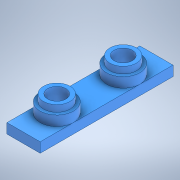
# Autodesk Inventor part: 4mm_Roller_Spacer
Saved by Autodesk Inventor 2021 (Build 250183000, 183)
## iProperties
Created: 2021-03-29
Part Number: 4mm_Roller_Spacer
Material: PET Plastic
Document SubType Name: Modeling
Designer: Jorian Brusind
Density: 1.541 g/cm^3
Appearance: Cyan
Author: Jorian Brusind
Autodesk Inventor part; units mm, degrees
ref_plane "YZ Plane" through (0, 0, 0) normal (1, 0, 0) x (0, 1, 0)
ref_plane "XZ Plane" through (0, 0, 0) normal (0, 1, 0) x (-1, 0, 0)
ref_plane "XY Plane" through (0, 0, 0) normal (0, 0, 1) x (1, 0, 0)
sketch "Sketch1" plane through (0, 0, 0) normal (0, 1, 0) x (-1, 0, 0)
  line L0 (0, 0) -> (10, 0)
  line L1 (10, 0) -> (10, -40)
  line L2 (10, -40) -> (0, -40)
  line L3 (0, -40) -> (0, 0)
  circle A0 centre (5, -10) radius 2.75
  circle A1 centre (5, -30) radius 2.75
  dimension "d0" = 10
  dimension "d1" = 40
  dimension "d2" = 5.5
  dimension "d3" = 5.5
  dimension "d4" = 10
  dimension "d5" = 10
  dimension "d6" = 5
  constraints: 8 end point, 2 centre point, 2 parallel, 1 horizontal, 1 perpendicular, 1 vertical alignment
  measures "d0" distance of L1.end L2.end
  measures "d1" distance of L0.end L1.end
  measures "d2" diameter of A0
  measures "d3" diameter of A1
  measures "d4" distance from line of L2 A1.centre
  measures "d5" distance from line of L0 A0.centre
  measures "d6" distance from line of L1 A0.centre
extrude "Extrusion1" add sketch "Sketch1" along normal blind 3
sketch "Sketch2" plane through (0, 3, 0) normal (0, 1, 0) x (1, 0, 0)
  circle A0 centre (-5, 10) radius 2.75 projected
  circle A1 centre (-5, 10) radius 2.75
  circle A2 centre (-5, 10) radius 4
  circle A3 centre (-5, 30) radius 2.75 projected
  circle A4 centre (-5, 30) radius 2.75
  circle A5 centre (-5, 30) radius 4
  point P0 (0, 0)
  dimension "d9" = 5.5
  dimension "d10" = 8
  dimension "d11" = 5.5
  dimension "d12" = 8
  constraints: 4 centre point, 4 coincident
  measures "d9" diameter of A1
  measures "d10" diameter of A2
  measures "d11" diameter of A4
  measures "d12" diameter of A5
extrude "Extrusion2" add sketch "Sketch2" along normal blind 5
sketch "Sketch3" plane through (0, 3, 0) normal (0, 1, 0) x (1, 0, 0)
  circle A0 centre (-5, 10) radius 2.75 projected
  circle A1 centre (-5, 10) radius 4
  circle A2 centre (-5, 10) radius 5
  circle A3 centre (-5, 30) radius 2.75 projected
  circle A4 centre (-5, 30) radius 2.75
  circle A5 centre (-5, 30) radius 5
  point P0 (0, 0)
  dimension "d15" = 10
  dimension "d16" = 10
  constraints: 4 centre point, 4 coincident
  measures "d15" diameter of A2
  measures "d16" diameter of A5
extrude "Extrusion3" add sketch "Sketch3" along normal blind 3 contours A2 | A5
body "Solid1"
